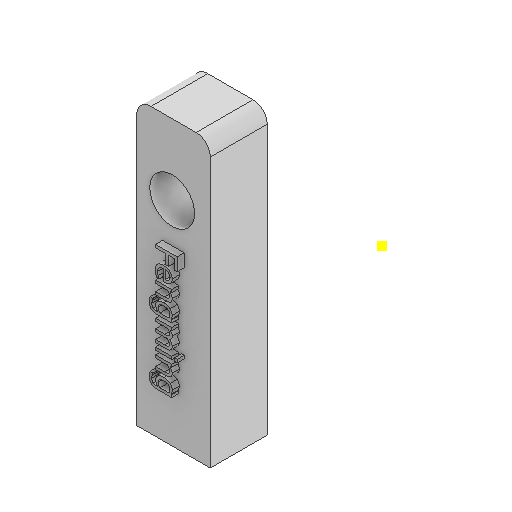
# Autodesk Inventor part: fengmingbodyplayer
Saved by Autodesk Inventor 2025 (Build 290162000, 162)
## iProperties
Created: 2024-11-17
Part Number: fengmingbodyplayer
Material: Generic
Document SubType Name: Modeling
Designer: wj
Density: 1 g/cm^3
Appearance: Default
Author: wj
Autodesk Inventor part; units mm, degrees
ref_plane "YZ Plane" through (0, 0, 0) normal (1, 0, 0) x (0, 1, 0)
ref_plane "XZ Plane" through (0, 0, 0) normal (0, 1, 0) x (-1, 0, 0)
ref_plane "XY Plane" through (0, 0, 0) normal (0, 0, 1) x (1, 0, 0)
sketch "Sketch1" plane through (0, 0, 0) normal (0, 1, 0) x (-1, 0, 0)
  line L0 (7.4359, 13.2759) -> (-7.9392, 13.2759)
  line L1 (-7.9392, 13.2759) -> (-7.9392, -13.745)
  line L2 (-7.9392, -13.745) -> (7.4359, -13.745)
  line L3 (7.4359, -13.745) -> (7.4359, 13.2759)
  point P0 (0, 0)
  constraints: 8 end point, 2 parallel, 1 horizontal, 1 perpendicular
extrude "Extrusion1" add sketch "Sketch1" along normal blind 20
sketch "Sketch2" plane through (7.9392, 0, 13.2759) normal (1, 0, 0) x (0, 0, -1)
  point P0 (13.2759, 0)
sketch "Sketch3" plane through (7.9392, 0, -13.745) normal (0, 0, -1) x (-1, 0, 0)
  line L0 (0, 0) -> (15.3751, 0) projected
  line L1 (0, 20) -> (15.3751, 20)
  line L2 (15.3751, 20) -> (15.3751, 0)
  line L3 (15.3751, 0) -> (0, 0)
  line L4 (0, 0) -> (0, 20)
  point P0 (7.9392, 0)
  constraints: 8 end point, 2 parallel, 1 horizontal, 1 perpendicular
extrude "Extrusion2" cut sketch "Sketch3" against normal blind 25
fillet "Fillet1" radius 2 1 edges at (7.9392, 20, 12.2655)
fillet "Fillet2" radius 2 1 edges at (-7.4359, 20, 12.2655)
sketch "Sketch4" plane through (-7.4359, 0, 13.2759) normal (0, 0, 1) x (1, 0, 0)
  arc A0 (2, 20) -> (0, 18) centre (2, 18) ccw projected
  line L0 (0, 0) -> (0, 18) projected
  line L1 (0, 0) -> (15.3751, 0) projected
  line L2 (15.3751, 0) -> (15.3751, 18) projected
  arc A1 (15.3751, 18) -> (13.3751, 20) centre (13.3751, 18) ccw projected
  line L3 (2, 20) -> (13.3751, 20) projected
  point P0 (7.4359, 0)
extrude "Extrusion3" add sketch "Sketch4" along normal blind 6
sketch "Sketch5" plane through (7.9392, 0, 11.255) normal (1, 0, 0) x (0, 0, -1)
  line L0 (-8.0209, 18) -> (0, 18) projected
  line L1 (-8.0209, 0) -> (-8.0209, 18) projected
  line L2 (-8.0209, 0) -> (0, 0) projected
  line L3 (0, 0) -> (0, 18) projected
  line L4 (-8.0209, 20) -> (-8.0209, 18) projected
  line L5 (0, 0) -> (-8.0209, 0)
  line L6 (-8.0209, 0) -> (-8.0209, 20)
  line L7 (-8.0209, 20) -> (0, 20)
  line L8 (0, 20) -> (0, 0)
  point P0 (11.255, 0)
  constraints: 8 end point, 2 parallel, 1 horizontal, 1 perpendicular
extrude "Extrusion4" cut sketch "Sketch5" against normal blind 5
fillet "Fillet3" radius 2 1 edges at (2.9392, 20, 15.2655)
sketch "Sketch6" plane through (0, 0, 0) normal (0, -1, 0) x (1, 0, 0)
  line L0 (2.9392, 11.255) -> (2.9392, 19.2759) projected
  line L1 (-7.4359, 19.2759) -> (2.9392, 19.2759) projected
  line L2 (-7.4359, 11.255) -> (-7.4359, 19.2759) projected
  line L3 (-7.4359, 11.255) -> (2.9392, 11.255) projected
  point P0 (0, 0)
extrude "Extrusion5" add sketch "Sketch6" along normal blind 20
sketch "Sketch7" plane through (-7.4359, 0, 19.2759) normal (0, 0, 1) x (1, 0, 0)
  circle A0 centre (5, 10) radius 3.15
  line L0 (0, 18) -> (0, -20) projected
  line L1 (10.3751, -20) -> (0, -20) projected
  point P0 (7.4359, 0)
  point P1 (5.1876, -20)
  dimension "d13" = 6.3
  dimension "d14" = 5
  dimension "d15" = 30
  constraints: 1 centre point, 1 midpoint
  measures "d13" diameter of A0
  measures "d14" distance from line of L0 A0.centre
  measures "d15" vertical distance of point (5.188, -20) A0.centre
hole "Hole1" at (-2.4359, 10, 19.2759) direction (0, 0, -1) diameter 6.3 end through all
sketch "Sketch8" plane through (-7.4359, 0, 19.2759) normal (0, 0, 1) x (1, 0, 0)
  line L0 (6.7147, 4.7716) -> (6.7147, -0.696) construction
  line L1 (6.7147, -0.696) -> (-10.2418, -0.696) construction
  line L2 (-10.2418, -0.696) -> (-10.2418, 4.7716) construction
  line L3 (-10.2418, 4.7716) -> (6.7147, 4.7716) construction
  line L4 (6.3343, 2.64) -> (6.3343, 4.0578)
  line L5 (6.3343, 4.0578) -> (5.4747, 4.0578)
  line L6 (5.4747, 4.0578) -> (5.4747, 2.6993)
  line L7 (5.4747, 2.6993) -> (5.1141, 2.6993)
  line L8 (5.1141, 2.6993) -> (5.1141, 4.0578)
  line L9 (5.1141, 4.0578) -> (3.6469, 4.0578)
  line L10 (3.6469, 4.0578) -> (3.6469, 4.4629)
  line L11 (3.6469, 4.4629) -> (6.6949, 4.4629)
  line L12 (6.6949, 4.4629) -> (6.6949, 2.64)
  line L13 (6.6949, 2.64) -> (6.3343, 2.64)
  spline S0 degree 2 poles (3.5951, 1.3136) (3.5951, 1.862) (4.2101, 2.4646) (4.7782, 2.4646) knots 0 0 0 1 2 2 2
  spline S1 degree 2 poles (4.7782, 2.4646) (5.3364, 2.4646) (5.9984, 1.8792) (5.9984, 1.4075) knots 0 0 0 1 2 2 2
  spline S2 degree 2 poles (5.9984, 1.4075) (5.9984, 1.1951) (5.8749, 0.8665) (5.744, 0.7455) knots 0 0 0 1 2 2 2
  spline S3 degree 2 poles (5.744, 0.7455) (5.6131, 0.622) (5.2352, 0.4911) (4.961, 0.4911) knots 0 0 0 1 2 2 2
  line L14 (4.961, 0.4911) -> (4.751, 0.4911)
  line L15 (4.751, 0.4911) -> (4.751, 2.0744)
  spline S4 degree 2 poles (4.751, 2.0744) (4.3534, 2.0744) (3.931, 1.6742) (3.931, 1.3186) knots 0 0 0 1 2 2 2
  spline S5 degree 2 poles (3.931, 1.3186) (3.931, 1.1926) (3.9878, 0.9481) (4.0323, 0.8493) knots 0 0 0 1 2 2 2
  spline S6 degree 2 poles (4.0323, 0.8493) (4.0817, 0.7455) (4.1681, 0.6023) (4.2076, 0.5553) knots 0 0 0 1 2 2 2
  line L16 (4.2076, 0.5553) -> (4.2076, 0.5331)
  line L17 (4.2076, 0.5331) -> (3.7877, 0.5331)
  spline S7 degree 2 poles (3.7877, 0.5331) (3.7606, 0.5998) (3.6815, 0.8023) (3.6593, 0.8814) knots 0 0 0 1 2 2 2
  spline S8 degree 2 poles (3.6593, 0.8814) (3.6272, 0.9925) (3.5951, 1.1753) (3.5951, 1.3136) knots 0 0 0 1 2 2 2
  spline S9 degree 2 poles (5.045, 0.8665) (5.2006, 0.8715) (5.4278, 0.9357) (5.5044, 0.9975) knots 0 0 0 1 2 2 2
  spline S10 degree 2 poles (5.5044, 0.9975) (5.5908, 1.0641) (5.6822, 1.2741) (5.6822, 1.4297) knots 0 0 0 1 2 2 2
  spline S11 degree 2 poles (5.6822, 1.4297) (5.6822, 1.5828) (5.5908, 1.7977) (5.5019, 1.8867) knots 0 0 0 1 2 2 2
  spline S12 degree 2 poles (5.5019, 1.8867) (5.4105, 1.9731) (5.1907, 2.062) (5.045, 2.0744) knots 0 0 0 1 2 2 2
  line L18 (5.045, 2.0744) -> (5.045, 0.8665)
  line L19 (3.6469, -1.6949) -> (3.6469, -1.3095)
  line L20 (3.6469, -1.3095) -> (4.9511, -1.3095)
  spline S13 degree 2 poles (4.9511, -1.3095) (5.1092, -1.3095) (5.3809, -1.2799) (5.4624, -1.2354) knots 0 0 0 1 2 2 2
  spline S14 degree 2 poles (5.4624, -1.2354) (5.5488, -1.1885) (5.6328, -1.0205) (5.6328, -0.8773) knots 0 0 0 1 2 2 2
  spline S15 degree 2 poles (5.6328, -0.8773) (5.6328, -0.734) (5.4797, -0.4302) (5.3562, -0.2845) knots 0 0 0 1 2 2 2
  line L21 (5.3562, -0.2845) -> (3.6469, -0.2845)
  line L22 (3.6469, -0.2845) -> (3.6469, 0.1008)
  line L23 (3.6469, 0.1008) -> (5.9342, 0.1008)
  line L24 (5.9342, 0.1008) -> (5.9342, -0.2845)
  line L25 (5.9342, -0.2845) -> (5.6798, -0.2845)
  spline S16 degree 2 poles (5.6798, -0.2845) (5.8354, -0.4574) (5.9984, -0.7908) (5.9984, -0.9786) knots 0 0 0 1 2 2 2
  spline S17 degree 2 poles (5.9984, -0.9786) (5.9984, -1.3145) (5.5538, -1.6949) (5.1314, -1.6949) knots 0 0 0 1 2 2 2
  line L26 (5.1314, -1.6949) -> (3.6469, -1.6949)
  spline S18 degree 2 poles (3.2814, -2.3173) (3.2641, -2.3568) (3.2097, -2.5075) (3.1875, -2.6038) knots 0 0 0 1 2 2 2
  spline S19 degree 2 poles (3.1875, -2.6038) (3.1603, -2.71) (3.1282, -2.8904) (3.1282, -2.9966) knots 0 0 0 1 2 2 2
  spline S20 degree 2 poles (3.1282, -2.9966) (3.1282, -3.1744) (3.2221, -3.4214) (3.3061, -3.4906) knots 0 0 0 1 2 2 2
  spline S21 degree 2 poles (3.3061, -3.4906) (3.39, -3.5573) (3.6099, -3.6091) (3.7507, -3.6091) knots 0 0 0 1 2 2 2
  line L27 (3.7507, -3.6091) -> (3.9507, -3.6091)
  spline S22 degree 2 poles (3.9507, -3.6091) (3.8149, -3.4535) (3.6865, -3.1546) (3.6865, -2.9299) knots 0 0 0 1 2 2 2
  spline S23 degree 2 poles (3.6865, -2.9299) (3.6865, -2.5396) (4.2669, -2.0777) (4.8128, -2.0777) knots 0 0 0 1 2 2 2
  spline S24 degree 2 poles (4.8128, -2.0777) (5.0968, -2.0777) (5.5365, -2.2383) (5.6921, -2.3716) knots 0 0 0 1 2 2 2
  spline S25 degree 2 poles (5.6921, -2.3716) (5.8378, -2.5001) (5.9984, -2.8533) (5.9984, -3.041) knots 0 0 0 1 2 2 2
  spline S26 degree 2 poles (5.9984, -3.041) (5.9984, -3.2189) (5.9144, -3.4782) (5.8378, -3.6091) knots 0 0 0 1 2 2 2
  line L28 (5.8378, -3.6091) -> (5.9342, -3.6314)
  line L29 (5.9342, -3.6314) -> (5.9342, -3.9944)
  line L30 (5.9342, -3.9944) -> (3.9088, -3.9944)
  spline S27 degree 2 poles (3.9088, -3.9944) (3.3258, -3.9944) (2.7824, -3.4881) (2.7824, -2.9669) knots 0 0 0 1 2 2 2
  spline S28 degree 2 poles (2.7824, -2.9669) (2.7824, -2.799) (2.8368, -2.4482) (2.8812, -2.2975) knots 0 0 0 1 2 2 2
  line L31 (2.8812, -2.2975) -> (3.2814, -2.2975)
  line L32 (3.2814, -2.2975) -> (3.2814, -2.3173)
  line L33 (4.2669, -3.6091) -> (5.5241, -3.6091)
  spline S29 degree 2 poles (5.5241, -3.6091) (5.5933, -3.4659) (5.6526, -3.2238) (5.6526, -3.1028) knots 0 0 0 1 2 2 2
  spline S30 degree 2 poles (5.6526, -3.1028) (5.6526, -2.8113) (5.2228, -2.4754) (4.8202, -2.4754) knots 0 0 0 1 2 2 2
  spline S31 degree 2 poles (4.8202, -2.4754) (4.4398, -2.4754) (4.0421, -2.7298) (4.0421, -3.0163) knots 0 0 0 1 2 2 2
  spline S32 degree 2 poles (4.0421, -3.0163) (4.0421, -3.167) (4.1607, -3.4832) (4.2669, -3.6091) knots 0 0 0 1 2 2 2
  line L34 (3.6469, -7.1462) -> (4.9709, -7.1462)
  spline S33 degree 2 poles (4.9709, -7.1462) (5.1289, -7.1462) (5.3982, -7.1215) (5.4723, -7.082) knots 0 0 0 1 2 2 2
  spline S34 degree 2 poles (5.4723, -7.082) (5.5538, -7.0424) (5.6328, -6.8918) (5.6328, -6.7609) knots 0 0 0 1 2 2 2
  spline S35 degree 2 poles (5.6328, -6.7609) (5.6328, -6.6423) (5.4871, -6.3706) (5.3488, -6.2273) knots 0 0 0 1 2 2 2
  spline S36 degree 2 poles (5.3488, -6.2273) (5.3142, -6.2298) (5.2179, -6.2348) (5.1536, -6.2348) knots 0 0 0 1 2 2 2
  line L35 (5.1536, -6.2348) -> (3.6469, -6.2348)
  line L36 (3.6469, -6.2348) -> (3.6469, -5.8494)
  line L37 (3.6469, -5.8494) -> (4.9709, -5.8494)
  spline S37 degree 2 poles (4.9709, -5.8494) (5.1289, -5.8494) (5.3982, -5.8247) (5.4723, -5.7852) knots 0 0 0 1 2 2 2
  spline S38 degree 2 poles (5.4723, -5.7852) (5.5538, -5.7457) (5.6328, -5.595) (5.6328, -5.4641) knots 0 0 0 1 2 2 2
  spline S39 degree 2 poles (5.6328, -5.4641) (5.6328, -5.3406) (5.4772, -5.0664) (5.3562, -4.938) knots 0 0 0 1 2 2 2
  line L38 (5.3562, -4.938) -> (3.6469, -4.938)
  line L39 (3.6469, -4.938) -> (3.6469, -4.5527)
  line L40 (3.6469, -4.5527) -> (5.9342, -4.5527)
  line L41 (5.9342, -4.5527) -> (5.9342, -4.938)
  line L42 (5.9342, -4.938) -> (5.6822, -4.938)
  spline S40 degree 2 poles (5.6822, -4.938) (5.8329, -5.0887) (5.9984, -5.3851) (5.9984, -5.5629) knots 0 0 0 1 2 2 2
  spline S41 degree 2 poles (5.9984, -5.5629) (5.9984, -5.7655) (5.8131, -6.0791) (5.6032, -6.1607) knots 0 0 0 1 2 2 2
  spline S42 degree 2 poles (5.6032, -6.1607) (5.7983, -6.336) (5.9984, -6.667) (5.9984, -6.8597) knots 0 0 0 1 2 2 2
  spline S43 degree 2 poles (5.9984, -6.8597) (5.9984, -7.0079) (5.907, -7.2499) (5.8033, -7.3389) knots 0 0 0 1 2 2 2
  spline S44 degree 2 poles (5.8033, -7.3389) (5.6995, -7.4302) (5.3883, -7.5315) (5.1536, -7.5315) knots 0 0 0 1 2 2 2
  line L43 (5.1536, -7.5315) -> (3.6469, -7.5315)
  line L44 (3.6469, -7.5315) -> (3.6469, -7.1462)
  line L45 (3.6469, -8.4652) -> (3.6469, -8.0799)
  line L46 (3.6469, -8.0799) -> (5.9342, -8.0799)
  line L47 (5.9342, -8.0799) -> (5.9342, -8.4652)
  line L48 (5.9342, -8.4652) -> (3.6469, -8.4652)
  line L49 (6.3145, -8.4923) -> (6.3145, -8.0552)
  line L50 (6.3145, -8.0552) -> (6.7147, -8.0552)
  line L51 (6.7147, -8.0552) -> (6.7147, -8.4923)
  line L52 (6.7147, -8.4923) -> (6.3145, -8.4923)
  line L53 (3.6469, -10.8265) -> (3.6469, -10.4412)
  line L54 (3.6469, -10.4412) -> (4.9511, -10.4412)
  spline S45 degree 2 poles (4.9511, -10.4412) (5.1092, -10.4412) (5.3809, -10.4116) (5.4624, -10.3671) knots 0 0 0 1 2 2 2
  spline S46 degree 2 poles (5.4624, -10.3671) (5.5488, -10.3202) (5.6328, -10.1522) (5.6328, -10.0089) knots 0 0 0 1 2 2 2
  spline S47 degree 2 poles (5.6328, -10.0089) (5.6328, -9.8657) (5.4797, -9.5619) (5.3562, -9.4161) knots 0 0 0 1 2 2 2
  line L55 (5.3562, -9.4161) -> (3.6469, -9.4161)
  line L56 (3.6469, -9.4161) -> (3.6469, -9.0308)
  line L57 (3.6469, -9.0308) -> (5.9342, -9.0308)
  line L58 (5.9342, -9.0308) -> (5.9342, -9.4161)
  line L59 (5.9342, -9.4161) -> (5.6798, -9.4161)
  spline S48 degree 2 poles (5.6798, -9.4161) (5.8354, -9.589) (5.9984, -9.9225) (5.9984, -10.1102) knots 0 0 0 1 2 2 2
  spline S49 degree 2 poles (5.9984, -10.1102) (5.9984, -10.4461) (5.5538, -10.8265) (5.1314, -10.8265) knots 0 0 0 1 2 2 2
  line L60 (5.1314, -10.8265) -> (3.6469, -10.8265)
  spline S50 degree 2 poles (3.2814, -11.449) (3.2641, -11.4885) (3.2097, -11.6391) (3.1875, -11.7355) knots 0 0 0 1 2 2 2
  spline S51 degree 2 poles (3.1875, -11.7355) (3.1603, -11.8417) (3.1282, -12.022) (3.1282, -12.1282) knots 0 0 0 1 2 2 2
  spline S52 degree 2 poles (3.1282, -12.1282) (3.1282, -12.3061) (3.2221, -12.5531) (3.3061, -12.6222) knots 0 0 0 1 2 2 2
  spline S53 degree 2 poles (3.3061, -12.6222) (3.39, -12.6889) (3.6099, -12.7408) (3.7507, -12.7408) knots 0 0 0 1 2 2 2
  line L61 (3.7507, -12.7408) -> (3.9507, -12.7408)
  spline S54 degree 2 poles (3.9507, -12.7408) (3.8149, -12.5852) (3.6865, -12.2863) (3.6865, -12.0615) knots 0 0 0 1 2 2 2
  spline S55 degree 2 poles (3.6865, -12.0615) (3.6865, -11.6713) (4.2669, -11.2094) (4.8128, -11.2094) knots 0 0 0 1 2 2 2
  spline S56 degree 2 poles (4.8128, -11.2094) (5.0968, -11.2094) (5.5365, -11.3699) (5.6921, -11.5033) knots 0 0 0 1 2 2 2
  spline S57 degree 2 poles (5.6921, -11.5033) (5.8378, -11.6317) (5.9984, -11.985) (5.9984, -12.1727) knots 0 0 0 1 2 2 2
  spline S58 degree 2 poles (5.9984, -12.1727) (5.9984, -12.3505) (5.9144, -12.6099) (5.8378, -12.7408) knots 0 0 0 1 2 2 2
  line L62 (5.8378, -12.7408) -> (5.9342, -12.763)
  line L63 (5.9342, -12.763) -> (5.9342, -13.1261)
  line L64 (5.9342, -13.1261) -> (3.9088, -13.1261)
  spline S59 degree 2 poles (3.9088, -13.1261) (3.3258, -13.1261) (2.7824, -12.6197) (2.7824, -12.0986) knots 0 0 0 1 2 2 2
  spline S60 degree 2 poles (2.7824, -12.0986) (2.7824, -11.9306) (2.8368, -11.5799) (2.8812, -11.4292) knots 0 0 0 1 2 2 2
  line L65 (2.8812, -11.4292) -> (3.2814, -11.4292)
  line L66 (3.2814, -11.4292) -> (3.2814, -11.449)
  line L67 (4.2669, -12.7408) -> (5.5241, -12.7408)
  spline S61 degree 2 poles (5.5241, -12.7408) (5.5933, -12.5975) (5.6526, -12.3555) (5.6526, -12.2344) knots 0 0 0 1 2 2 2
  spline S62 degree 2 poles (5.6526, -12.2344) (5.6526, -11.943) (5.2228, -11.607) (4.8202, -11.607) knots 0 0 0 1 2 2 2
  spline S63 degree 2 poles (4.8202, -11.607) (4.4398, -11.607) (4.0421, -11.8615) (4.0421, -12.148) knots 0 0 0 1 2 2 2
  spline S64 degree 2 poles (4.0421, -12.148) (4.0421, -12.2986) (4.1607, -12.6148) (4.2669, -12.7408) knots 0 0 0 1 2 2 2
  point P0 (7.4359, 0)
  constraints: 2 other
extrude "Extrusion6" add sketch "Sketch8" along normal blind 1
body "Solid1"
